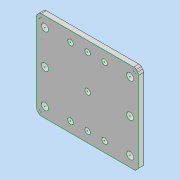
# Autodesk Inventor part: Diode_laser_Mount
Saved by Autodesk Inventor 2020 (Build 240168000, 168)
## iProperties
Created: 2021-07-14
Part Number: Diode_laser_Mount
Material: 一般
Document SubType Name: Modeling
Designer: ken113
Density: 1 g/cm^3
Appearance: 既定
Author: ken113
Autodesk Inventor part; units mm, degrees
ref_plane "YZ Plane" through (0, 0, 0) normal (1, 0, 0) x (0, 1, 0)
ref_plane "XZ Plane" through (0, 0, 0) normal (0, 1, 0) x (-1, 0, 0)
ref_plane "XY Plane" through (0, 0, 0) normal (0, 0, 1) x (1, 0, 0)
sketch "スケッチ1" plane through (0, 0, 0) normal (0, 0, 1) x (1, 0, 0)
  line L0 (30, -26) -> (-30, -26)
  line L1 (-30, -26) -> (-30, 26)
  line L2 (-30, 26) -> (30, 26)
  line L3 (30, 26) -> (30, -26)
  line L4 (30, -26) -> (-30, 26) construction
  line L5 (-30, -26) -> (30, 26) construction
  point P0 (0, 0)
  dimension "d0" = 60
  dimension "d1" = 52
  constraints: 12 end point, 2 midpoint, 2 parallel, 1 horizontal, 1 perpendicular
  measures "d0" distance of L1.end L2.end
  measures "d1" distance of L0.end L1.end
extrude "押し出し1" add sketch "スケッチ1" along normal blind 3
sketch "スケッチ2" plane through (0, 0, 3) normal (0, 0, 1) x (1, 0, 0)
  line L0 (-10, -20) -> (10, -20)
  line L1 (10, -20) -> (10, 20)
  line L2 (10, 20) -> (-10, 20)
  line L3 (-10, 20) -> (-10, -20)
  line L4 (-10, -20) -> (10, 20) construction
  line L5 (10, -20) -> (-10, 20) construction
  line L6 (-30, -26) -> (30, -26) projected
  point P0 (0, 0)
  point P1 (0, 20)
  point P2 (0, -20)
  dimension "d4" = 20
  dimension "d5" = 40
  dimension "d6" = 6
  constraints: 12 end point, 3 midpoint, 2 parallel, 1 horizontal, 1 perpendicular
  measures "d4" distance of L2.end L1.end
  measures "d5" distance of L1.end L0.end
  measures "d6" distance between parallel lines of L0 L6
hole "穴1" at (-10, 20, 3) at (-10, -20, 3) at (10, -20, 3) at (10, 20, 3) at (0, -20, 3) at (0, 0, 3) at (0, 20, 3) direction (0, 0, -1) diameter 3.3 depth 8.8
sketch "スケッチ4" plane through (0, 0, 3) normal (0, 0, 1) x (1, 0, 0)
  line L0 (-25, -20) -> (25, -20)
  line L1 (25, -20) -> (25, 20)
  line L2 (25, 20) -> (-25, 20)
  line L3 (-25, 20) -> (-25, -20)
  line L4 (-25, -20) -> (25, 20) construction
  line L5 (25, -20) -> (-25, 20) construction
  point P0 (0, 0)
  point P1 (0, 20)
  point P2 (0, -20)
  point P3 (0, 0)
  point P4 (-25, 0)
  point P5 (25, 0)
  dimension "d14" = 50
  dimension "d15" = 40
  constraints: 12 end point, 6 midpoint, 2 parallel, 1 coincident, 1 horizontal, 1 perpendicular
  measures "d14" distance of L2.end L1.end
  measures "d15" distance of L1.end L0.end
hole "穴2" at (-25, 20, 3) at (-25, -20, 3) at (25, -20, 3) at (25, 20, 3) at (-25, 0, 3) at (25, 0, 3) direction (0, 0, -1) diameter 4.2 depth 8.8
chamfer "面取り1" distance 2 angle 45 4 edges at (-30, 26, 1.5) (-30, -26, 1.5) (30, -26, 1.5) (30, 26, 1.5)
fillet "フィレット2" radius 2 6 edges at (30, 24, 1.5) (28, 26, 1.5) (-28, 26, 1.5) (-30, 24, 1.5) (-30, -24, 1.5) (-28, -26, 1.5)
sketch "スケッチ5" plane through (0, 0, 3) normal (0, 0, 1) x (1, 0, 0)
  circle A0 centre (-25, 0) radius 2.1 projected
  circle A1 centre (25, -20) radius 2.1 projected
  circle A2 centre (-25, 20) radius 2.1 projected
  circle A3 centre (-25, -20) radius 2.1 projected
  circle A4 centre (25, 20) radius 2.1 projected
  circle A5 centre (25, 0) radius 2.1 projected
  circle A6 centre (0, 0) radius 1.65 projected
  circle A7 centre (10, 20) radius 1.65 projected
  circle A8 centre (-10, -20) radius 1.65 projected
  circle A9 centre (-10, 20) radius 1.65 projected
  circle A10 centre (10, -20) radius 1.65 projected
  circle A11 centre (0, -20) radius 1.65 projected
  circle A12 centre (0, 20) radius 1.65 projected
  arc A13 (-28.5858, -25.4142) -> (-27.1716, -26) centre (-27.1716, -24) ccw projected
  line L0 (-27.1716, -26) -> (28, -26) projected
  line L1 (30, -24) -> (28, -26) projected
  line L2 (30, -24) -> (30, 23.1716) projected
  arc A14 (30, 23.1716) -> (29.4142, 24.5858) centre (28, 23.1716) ccw projected
  line L3 (28.5858, 25.4142) -> (29.4142, 24.5858) projected
  arc A15 (28.5858, 25.4142) -> (27.1716, 26) centre (27.1716, 24) ccw projected
  line L4 (27.1716, 26) -> (-27.1716, 26) projected
  arc A16 (-27.1716, 26) -> (-28.5858, 25.4142) centre (-27.1716, 24) ccw projected
  line L5 (-29.4142, 24.5858) -> (-28.5858, 25.4142) projected
  arc A17 (-29.4142, 24.5858) -> (-30, 23.1716) centre (-28, 23.1716) ccw projected
  line L6 (-30, 23.1716) -> (-30, -23.1716) projected
  arc A18 (-30, -23.1716) -> (-29.4142, -24.5858) centre (-28, -23.1716) ccw projected
  line L7 (-28.5858, -25.4142) -> (-29.4142, -24.5858) projected
  point P0 (0, 0)
